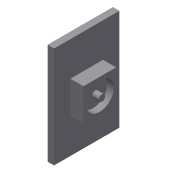
# Autodesk Inventor part: 00_LED_neopixel_single
Saved by Autodesk Inventor 2019.4 (Build 234330000, 330)
## iProperties
Created: 2021-02-25
Part Number: 00_LED_neopixel_single
Material: Generic
Document SubType Name: Modeling
Designer: diederichbenedict
Density: 1 g/cm^3
Appearance: Default
Author: diederichbenedict
Autodesk Inventor part; units mm, degrees
ref_plane "YZ Plane" through (0, 0, 0) normal (1, 0, 0) x (0, 1, 0)
ref_plane "XZ Plane" through (0, 0, 0) normal (0, 1, 0) x (-1, 0, 0)
ref_plane "XY Plane" through (0, 0, 0) normal (0, 0, 1) x (1, 0, 0)
sketch "Sketch1" plane through (0, 0, 0) normal (1, 0, 0) x (0, 1, 0)
  line L0 (-7.75, -5) -> (7.75, -5)
  line L1 (7.75, -5) -> (7.75, 5)
  line L2 (7.75, 5) -> (-7.75, 5)
  line L3 (-7.75, 5) -> (-7.75, -5)
  line L4 (-7.75, -5) -> (7.75, 5) construction
  line L5 (7.75, -5) -> (-7.75, 5) construction
  point P0 (0, 0)
  dimension "d0" = 15.5
  dimension "d1" = 10
  constraints: 12 end point, 2 midpoint, 2 parallel, 1 horizontal, 1 perpendicular
  measures "d0" distance of L2.end L1.end
  measures "d1" distance of L1.end L0.end
extrude "Extrusion1" add sketch "Sketch1" along normal blind 1
sketch "Sketch2" plane through (1, 0, 0) normal (1, 0, 0) x (0, 0, -1)
  line L0 (-2.5, 2.5) -> (2.5, 2.5)
  line L1 (2.5, 2.5) -> (2.5, -2.5)
  line L2 (2.5, -2.5) -> (-2.5, -2.5)
  line L3 (-2.5, -2.5) -> (-2.5, 2.5)
  line L4 (-2.5, 2.5) -> (2.5, -2.5) construction
  line L5 (2.5, 2.5) -> (-2.5, -2.5) construction
  point P0 (0, 0)
  dimension "d4" = 5
  dimension "d5" = 5
  constraints: 12 end point, 2 midpoint, 2 parallel, 1 horizontal, 1 perpendicular
  measures "d4" distance of L1.end L2.end
  measures "d5" distance of L0.end L1.end
extrude "Extrusion2" add sketch "Sketch2" along normal blind 2
sketch "Sketch3" plane through (3, 0, 0) normal (1, 0, 0) x (0, 0, -1)
  line L0 (2.5, 2.5) -> (-2.5, 2.5) projected
  line L1 (-2.5, 2.5) -> (-2.5, -2.5) projected
  line L2 (-2.5, -2.5) -> (2.5, -2.5) projected
  line L3 (2.5, -2.5) -> (2.5, 2.5) projected
  circle A0 centre (0, 0) radius 2.1413
  circle A1 centre (0, 0) radius 0.3761
  constraints: 2 centre point, 2 coincident
extrude "Extrusion3" cut sketch "Sketch3" against normal blind 1 contours A0
sketch "Sketch4" plane through (3, 0, 2.362) normal (1, 0, 0) x (0, 1, 0)
  circle A0 centre (0, -2.362) radius 0.3761 projected
extrude "Extrusion4" add sketch "Sketch4" along normal blind 15
body "Solid1"
